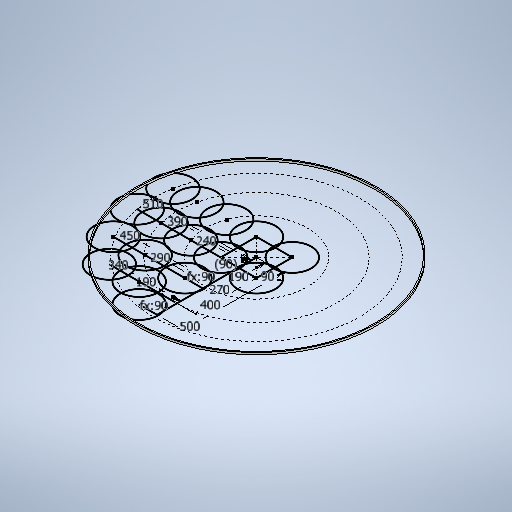
# Autodesk Inventor part: TZS 1759 DIM filter-distribution-system 1200
Saved by Autodesk Inventor 2025.1 (Build 291241020, 241B)
## iProperties
Created: 2025-06-24
Part Number: TZS 1759 DIM filter-distribution-system 1200
Material: Generic
Document SubType Name: Modeling
Designer: user
Density: 1 g/cm^3
Appearance: Default
Sheet Metal Rule: Default
way_tube_L5: 120.000 mm
way_tube_L6: 90.000 mm
way_tube_L7: 20.000 mm
way_tube_L8: 90.000 mm
way_tube_L9: 80.000 mm
way_tube_L10: 80.000 mm
Author: user
Autodesk Inventor part; units mm, degrees
ref_plane "YZ Plane" through (0, 0, 0) normal (1, 0, 0) x (0, 1, 0)
ref_plane "XZ Plane" through (0, 0, 0) normal (0, 1, 0) x (-1, 0, 0)
ref_plane "XY Plane" through (0, 0, 0) normal (0, 0, 1) x (1, 0, 0)
sketch "Sketch1" plane through (0, 0, 0) normal (0, 0, 1) x (1, 0, 0)
  circle A0 centre (0, 0) radius 600
  circle A1 centre (0, 0) radius 594
  dimension "d0" = 1200
  dimension "d1" = 6
  constraints: 2 centre point, 1 coincident
  measures "d0" diameter of A0
  measures "d1" radial gap between concentric circles of A0 A1
extrude "Extrusion1" add sketch "Sketch1" along normal blind 10
sketch "Sketch2" plane through (0, 0, 0) normal (0, 0, 1) x (1, 0, 0)
  circle A0 centre (0, 0) radius 517.8803 construction
  circle A1 centre (0, 0) radius 400.2499 construction
  circle A2 centre (0, 0) radius 256.3201 construction
  circle A3 centre (90, -90) radius 95
  circle A4 centre (-90, -90) radius 95
  circle A5 centre (-90, 90) radius 95
  circle A6 centre (90, 90) radius 95
  line L0 (90, 90) -> (-90, 90)
  line L1 (-90, 90) -> (-90, -90)
  line L2 (-90, -90) -> (90, -90)
  line L3 (90, -90) -> (90, 90)
  line L4 (90, 90) -> (-90, -90) construction
  line L5 (-90, 90) -> (90, -90) construction
  circle A7 centre (-240, -90) radius 95
  circle A8 centre (-390, -90) radius 95
  circle A9 centre (-510, -90) radius 95
  circle A10 centre (-90, -270) radius 95
  circle A11 centre (-90, -500) radius 95
  circle A12 centre (-290, -270) radius 95
  circle A13 centre (-450, -270) radius 95
  circle A14 centre (-340, -400) radius 95
  circle A15 centre (-240, 90) radius 95
  circle A16 centre (-390, 90) radius 95
  circle A17 centre (-510, 90) radius 95
  line L6 (-90, -90) -> (-510, -90)
  line L7 (0, 0) -> (0, -500)
  line L8 (0, -500) -> (-90, -500)
  line L9 (0, -400) -> (-340, -400)
  line L10 (0, -270) -> (-450, -270)
  circle A18 centre (-190, -400) radius 95
  dimension "d4" = 190
  dimension "d7" = 90
  dimension "d8" = 270
  dimension "d9" = 400
  dimension "d10" = 500
  dimension "d11" = 240
  dimension "d12" = 390
  dimension "d13" = 510
  dimension "d14" = 90
  dimension "d15" = 90
  dimension "d16" = 290
  dimension "d17" = 450
  dimension "d18" = 190
  dimension "d19" = 340
  dimension "d20" = 90
  constraints: 22 end point, 19 centre point, 15 equal radius, 11 point on line, 7 coincident, 6 perpendicular, 6 point on circle, 2 horizontal, 2 midpoint, 2 parallel
  measures "d4" diameter of A3
  measures "d7" distance from line of L2 point (0, 0)
  measures "d8" distance from line of L10 point (0, 0)
  measures "d9" distance from line of point (0, 0) L9
  measures "d10" distance from line of L8 point (0, 0)
  measures "d11" horizontal distance of A7.centre point (0, 0)
  measures "d12" horizontal distance of A8.centre point (0, 0)
  measures "d13" distance from line of L6.end L7
  measures "d14" distance from line of L7 A10.centre
  measures "d15" distance of L7.end L8.end
  measures "d16" distance from line of L7 A12.centre
  measures "d17" distance from line of L7 A13.centre
  measures "d18" distance from line of A18.centre L7
  measures "d19" distance of L9.start L9.end
  measures "d20" distance from line of L7 L1.end
sketch "Sketch3" plane through (0, 0, 0) normal (0, 0, 1) x (1, 0, 0)
  circle A0 centre (-104.0992, -233.3488) radius 95
  circle A1 centre (-161.9131, -395.3117) radius 95
  circle A2 centre (-91.7953, -514.3257) radius 95
  circle A3 centre (-280.9346, -260.412) radius 95
  circle A4 centre (-299.5406, -418.8761) radius 95
  circle A5 centre (-250.7395, 99.5106) radius 95
  circle A6 centre (-395.8303, 87.9315) radius 95
  circle A7 centre (-535.2648, 91.0733) radius 95
  circle A8 centre (-460.3613, -287.8718) radius 95
  circle A9 centre (-531.2922, -111.9436) radius 95
  circle A10 centre (-392.3143, -102.4845) radius 95
  circle A11 centre (0, 0) radius 542.9574 construction
  circle A12 centre (-253.2201, -93.0176) radius 95
  circle A13 centre (-90.4998, -81.9426) radius 95
  circle A14 centre (85.6841, -88.1302) radius 95
  circle A15 centre (-90.4998, 88.0537) radius 95
  circle A16 centre (0, 0) radius 405.4794 construction
  circle A17 centre (0, 0) radius 269.7641 construction
  circle A18 centre (85.6841, 88.0537) radius 95
  line L0 (0, 0) -> (0, -542.9574)
  line L1 (0, -75.783) -> (-531.2922, -111.9436)
  line L2 (0, -217.4173) -> (-460.3613, -287.8718)
  circle A19 centre (0, 0) radius 600
  line L3 (0, -367.5891) -> (-299.5406, -418.8761)
  line L4 (-91.7953, -514.3257) -> (0, -514.3257)
  point P0 (0, 0)
  dimension "d21" = 190
  dimension "d22" = 1200
  constraints: 20 centre point, 15 equal radius, 10 end point, 10 point on line, 8 point on circle, 5 coincident, 1 perpendicular, 1 vertical
  measures "d21" diameter of A14
  measures "d22" diameter of A19
equation "\"d14\" = d7"
equation "\"d15\" = d7"
equation "\"BendRadius\" = Thickness"
equation "\"BendReliefWidth\" = Thickness"
equation "\"BendReliefDepth\" = 0.5 * Thickness"
equation "\"CornerReliefSize\" = 4 * Thickness"
equation "\"MinimumRemnant\" = 2 * Thickness"
equation "\"TransitionRadius\" = BendRadius"
equation "\"JacobiRadiusSize\" = BendRadius"
equation "\"GapSize\" = Thickness"
equation "\"way_tube_L1\" = 1"
equation "\"way_tube_L2\" = 1"
equation "\"way_tube_L3\" = 1"
equation "\"way_tube_L4\" = 1"
equation "\"way_tube_L5\" = 120"
equation "\"way_tube_L6\" = 90"
equation "\"way_tube_L7\" = 20"
equation "\"way_tube_L8\" = 90"
equation "\"way_tube_L9\" = 80"
equation "\"way_tube_L10\" = 80"
equation "\"Thickness\" = 3.048"
body "Solid1"
